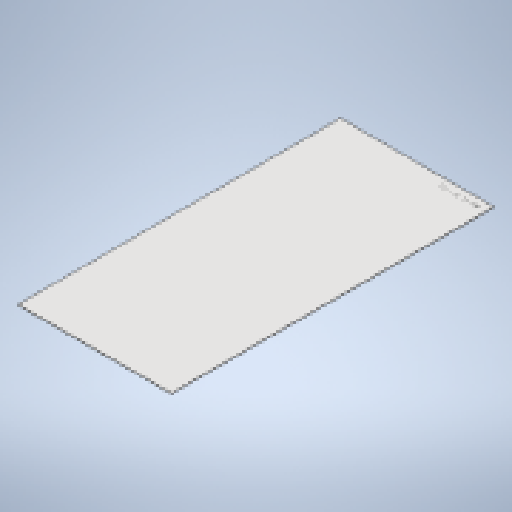
# Autodesk Inventor part: TRM 012 back main
Saved by Autodesk Inventor 2025 (Build 290162010, 162A)
## iProperties
Created: 2024-08-07
Part Number: TRM 012 back main
Material: AISI 304
Document SubType Name: Sheet Metal
Designer: pokla
Density: 8.02768 g/cm^3
Flat Pattern Width: 50 cm
Flat Pattern Length: 109.62 cm
Flat Pattern Area: 5481.01 cm^2
Sheet Metal Rule: AISI304 2mm Die16
Sheet Metal Width: 500,000 mm
Sheet Metal Length: 1096,202 mm
Sheet Metal Area: 548100,995 mm^2
Appearance: Default
Author: pokla
Autodesk Inventor part; units mm, degrees
ref_plane "YZ Plane" through (0, 0, 0) normal (1, 0, 0) x (0, 1, 0)
ref_plane "XZ Plane" through (0, 0, 0) normal (0, 1, 0) x (-1, 0, 0)
ref_plane "XY Plane" through (0, 0, 0) normal (0, 0, 1) x (1, 0, 0)
sketch "Sketch1" plane through (0, 0, 0) normal (0, 0, 1) x (1, 0, 0)
  line L0 (-250, -525) -> (250, -525)
  line L1 (250, -525) -> (250, 525)
  line L2 (250, 525) -> (-250, 525)
  line L3 (-250, 525) -> (-250, -525)
  line L4 (-250, -525) -> (250, 525) construction
  line L5 (250, -525) -> (-250, 525) construction
  point P0 (0, 0)
  dimension "d0" = 500
  dimension "d1" = 1050
  measures "d0" distance of L2.end L1.end
  measures "d1" distance of L1.end L0.end
extrude "Plate1" add sketch "Sketch1" along normal blind 2
sketch "Sketch2" plane through (0, 0, 0) normal (0, 0, -1) x (-1, 0, 0)
  line L0 (-230, 505) -> (-30, 505) construction
  line L1 (-30, 505) -> (-30, 485) construction
  line L2 (-30, 485) -> (-230, 485) construction
  line L3 (-230, 485) -> (-230, 505) construction
  line L4 (-250, 525) -> (250, 525) projected
  line L5 (-250, -525) -> (-250, 525) projected
  point P0 (0, 0)
  point P1 (-230, 495)
  dimension "d6" = 200
  dimension "d7" = 20
  dimension "d8" = 20
  dimension "d9" = 20
  constraints: 1 midpoint, 2 other
  measures "d6" distance of L0.start L0.end
  measures "d7" distance of L0.end L1.end
  measures "d8" distance between parallel lines of L4 L0
  measures "d9" distance from line of L5 point (-230, 495)
mark "Mark1"
sketch "Sketch3" plane through (250, -523, 0) normal (0, -1, 0) x (1, 0, 0)
  line L0 (-500, 0) -> (0, 0)
  line L1 (0, 0) -> (0, 50)
  line L2 (0, 50) -> (-500, 50)
  line L3 (-500, 50) -> (-500, 0)
  constraints: 6 end point, 1 horizontal, 1 perpendicular, 1 vertical
edge flange "Flange1" height 50 angle 90 thickness 2 bend radius 2.75 thickness toward (0, -1, 0) relief round relief width 2 relief depth 1 edges at (0, -525, 2) wall of the first edge with corners at (-250, -523, 0) (250, -523, 0) (250, -523, 50) (-250, -523, 50)
bend "Bend1"
corner "Corner1"
equation "\"d2\" = Thickness"
equation "\"d10\" = BendReliefWidth"
equation "\"d11\" = BendReliefDepth"
equation "\"d12\" = MinimumRemnant"
equation "\"d13\" = TransitionRadius"
equation "\"d16\" = BendRadius"
equation "\"d17\" = CornerReliefSize"
equation "\"d18\" = GapSize"
equation "\"d19\" = JacobiRadiusSize"
equation "\"BendReliefWidth\" = Thickness"
equation "\"BendReliefDepth\" = 0.5 * Thickness"
equation "\"CornerReliefSize\" = 4 * Thickness"
equation "\"MinimumRemnant\" = 2 * Thickness"
equation "\"TransitionRadius\" = BendRadius"
equation "\"JacobiRadiusSize\" = BendRadius"
equation "\"GapSize\" = Thickness"
equation "\"Thickness\" = 2"
equation "\"BendRadius\" = 2.75"
body "Solid1"
